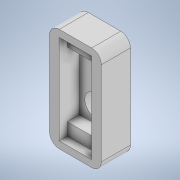
# Autodesk Inventor part: ramie03-5
Saved by Autodesk Inventor 2021 (Build 250183000, 183)
## iProperties
Created: 2021-11-08
Part Number: ramie03-5
Material: Generic
Document SubType Name: Modeling
Designer: Łukasz
Density: 1 g/cm^3
Appearance: Default
Author: Łukasz
Autodesk Inventor part; units mm, degrees
ref_plane "YZ Plane" through (0, 0, 0) normal (1, 0, 0) x (0, 1, 0)
ref_plane "XZ Plane" through (0, 0, 0) normal (0, 1, 0) x (-1, 0, 0)
ref_plane "XY Plane" through (0, 0, 0) normal (0, 0, 1) x (1, 0, 0)
sketch "Sketch1" plane through (0, 0, 0) normal (0, 0, 1) x (1, 0, 0)
  line L0 (0, 0) -> (-32, 0)
  line L1 (-32, 0) -> (-32, 64)
  line L2 (-32, 64) -> (0, 64)
  line L3 (0, 64) -> (0, 0)
  dimension "d0" = 32
  dimension "d1" = 64
  constraints: 8 end point, 2 parallel, 1 horizontal, 1 perpendicular
  measures "d0" distance of L1.end L2.end
  measures "d1" distance of L0.end L1.end
extrude "Extrusion1" add sketch "Sketch1" along normal blind 18
fillet "Fillet1" radius 6 4 edges at (0, 64, 9) (-32, 64, 9) (0, 0, 9) (-32, 0, 9)
sketch "Sketch2" plane through (0, 0, 18) normal (0, 0, 1) x (1, 0, 0)
  line L0 (-6, 52) -> (-26, 52)
  line L1 (-26, 52) -> (-26, 12)
  line L2 (-26, 12) -> (-6, 12)
  line L3 (-6, 12) -> (-6, 52)
  line L4 (-6, 64) -> (-26, 64) projected
  line L5 (0, 6) -> (0, 58) projected
  point P0 (0, 0)
  dimension "d5" = 20
  dimension "d6" = 40
  dimension "d7" = 12
  dimension "d8" = 6
  constraints: 8 end point, 2 parallel, 1 horizontal, 1 perpendicular
  measures "d5" distance of L2.end L1.end
  measures "d6" distance of L1.end L0.end
  measures "d7" distance between parallel lines of L4 L0
  measures "d8" distance between parallel lines of L5 L3
extrude "Extrusion2" cut sketch "Sketch2" against normal blind 12.5
sketch "Sketch3" plane through (0, 0, 5.5) normal (0, 0, 1) x (1, 0, 0)
  circle A0 centre (-16, 22) radius 6.75
  line L0 (-6, 52) -> (-6, 12) projected
  line L1 (-6, 12) -> (-26, 12) projected
  point P0 (0, 0)
  dimension "d11" = 13.5
  dimension "d12" = 10
  dimension "d13" = 10
  constraints: 1 centre point
  measures "d11" diameter of A0
  measures "d12" distance from line of L0 A0.centre
  measures "d13" distance from line of L1 A0.centre
extrude "Extrusion3" cut sketch "Sketch3" against normal up to surface (5.5 mm away)
sketch "Sketch4" plane through (0, 0, 18) normal (0, 0, 1) x (1, 0, 0)
  line L0 (-26, 52) -> (-6, 52) projected
  line L1 (-6, 52) -> (-26, 52)
  line L2 (-26, 52) -> (-26, 59.7)
  line L3 (-26, 59.7) -> (-6, 59.7)
  line L4 (-6, 59.7) -> (-6, 52)
  line L5 (-6, 12) -> (-26, 12) projected
  line L6 (-6, 12) -> (-26, 12)
  line L7 (-26, 12) -> (-26, 4.3)
  line L8 (-26, 4.3) -> (-6, 4.3)
  line L9 (-6, 4.3) -> (-6, 12)
  point P0 (0, 0)
  dimension "d16" = 7.7
  dimension "d17" = 20
  dimension "d18" = 7.7
  constraints: 16 end point, 4 parallel, 2 horizontal, 2 perpendicular
  measures "d16" distance of L1.end L2.end
  measures "d17" distance of L8.end L7.end
  measures "d18" distance of L7.end L6.end
extrude "Extrusion4" cut sketch "Sketch4" against normal blind 5
body "Solid1"
